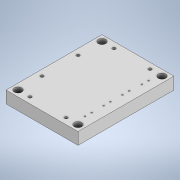
# Autodesk Inventor part: CasingBottomWithSlots
Saved by Autodesk Inventor 2020.4 (Build 244396010, 396A)
## iProperties
Created: 2021-10-02
Part Number: CasingBottomWithSlots
Material: Generic
Document SubType Name: Modeling
Designer: YUSTE
Density: 1 g/cm^3
Appearance: Default
Author: YUSTE
Autodesk Inventor part; units mm, degrees
ref_plane "YZ Plane" through (0, 0, 0) normal (1, 0, 0) x (0, 1, 0)
ref_plane "XZ Plane" through (0, 0, 0) normal (0, 1, 0) x (-1, 0, 0)
ref_plane "XY Plane" through (0, 0, 0) normal (0, 0, 1) x (1, 0, 0)
sketch "Sketch1" plane through (0, 0, 0) normal (0, 1, 0) x (-1, 0, 0)
  line L0 (0, 0) -> (152.4, 0)
  line L1 (152.4, 0) -> (152.4, 203.2)
  line L2 (152.4, 203.2) -> (0, 203.2)
  line L3 (0, 203.2) -> (0, 0)
  circle A0 centre (12.7, 190.5) radius 7.9375
  circle A1 centre (139.7, 190.5) radius 7.9375
  circle A2 centre (139.7, 12.7) radius 7.9375
  circle A3 centre (12.7, 12.7) radius 7.9375
  circle A4 centre (114.3, 190.5) radius 3.302
  circle A5 centre (38.1, 190.5) radius 3.302
  circle A6 centre (114.3, 12.7) radius 3.302
  circle A7 centre (38.1, 12.7) radius 3.302
  circle A8 centre (139.7, 139.7) radius 3.302
  circle A9 centre (139.7, 63.5) radius 3.302
  circle A10 centre (20.32, 168.148) radius 1.524
  circle A11 centre (20.32, 153.924) radius 1.524
  circle A12 centre (20.32, 128.524) radius 1.524
  circle A13 centre (20.32, 114.3) radius 1.524
  circle A14 centre (20.32, 88.9) radius 1.524
  circle A15 centre (20.32, 74.676) radius 1.524
  circle A16 centre (18.796, 49.276) radius 1.524
  circle A17 centre (18.796, 35.052) radius 1.524
  dimension "d0" = 152.4
  dimension "d1" = 203.2
  dimension "d40" = 15.875
  dimension "d41" = 15.875
  dimension "d42" = 15.875
  dimension "d43" = 15.875
  dimension "d44" = 12.7
  dimension "d45" = 12.7
  dimension "d46" = 12.7
  dimension "d47" = 12.7
  dimension "d48" = 12.7
  dimension "d49" = 12.7
  dimension "d50" = 12.7
  dimension "d51" = 12.7
  dimension "d52" = 177.8
  dimension "d53" = 127
  dimension "d54" = 6.604
  dimension "d55" = 6.604
  dimension "d56" = 25.4
  dimension "d57" = 25.4
  dimension "d58" = 12.7
  dimension "d59" = 12.7
  dimension "d60" = 6.604
  dimension "d61" = 6.604
  dimension "d62" = 12.7
  dimension "d63" = 12.7
  dimension "d64" = 25.4
  dimension "d65" = 25.4
  dimension "d66" = 6.604
  dimension "d67" = 6.604
  dimension "d68" = 50.8
  dimension "d69" = 50.8
  dimension "d70" = 12.7
  dimension "d71" = 12.7
  dimension "d72" = 3.048
  dimension "d73" = 3.048
  dimension "d74" = 3.048
  dimension "d75" = 3.048
  dimension "d76" = 3.048
  dimension "d77" = 3.048
  dimension "d78" = 20.32
  dimension "d79" = 20.32
  dimension "d80" = 20.32
  dimension "d81" = 20.32
  dimension "d82" = 20.32
  dimension "d83" = 20.32
  dimension "d84" = 22.352
  dimension "d85" = 14.224
  dimension "d86" = 25.4
  dimension "d87" = 14.224
  dimension "d88" = 25.4
  dimension "d89" = 14.224
  dimension "d90" = 3.048
  dimension "d91" = 3.048
  dimension "d92" = 25.4
  dimension "d93" = 14.224
  constraints: 18 centre point, 8 end point, 2 parallel, 1 horizontal, 1 perpendicular
  measures "d0" distance of L2.end L1.end
  measures "d1" distance of L1.end L0.end
  measures "d40" diameter of A0
  measures "d41" diameter of A1
  measures "d42" diameter of A2
  measures "d43" diameter of A3
  measures "d44" distance from line of L2 A0.centre
  measures "d45" distance from line of L3 A0.centre
  measures "d46" distance from line of L0 A3.centre
  measures "d47" distance from line of L3 A3.centre
  measures "d48" distance from line of L2 A1.centre
  measures "d49" distance from line of L1 A1.centre
  measures "d50" distance from line of L1 A2.centre
  measures "d51" distance from line of L0 A2.centre
  measures "d52" distance of A2.centre A1.centre
  measures "d53" distance of A0.centre A1.centre
  measures "d54" diameter of A4
  measures "d55" diameter of A5
  measures "d56" distance of A0.centre A5.centre
  measures "d57" distance of A1.centre A4.centre
  measures "d58" distance from line of L2 A4.centre
  measures "d59" distance from line of L2 A5.centre
  measures "d60" diameter of A6
  measures "d61" diameter of A7
  measures "d62" distance from line of L0 A7.centre
  measures "d63" distance from line of L0 A6.centre
  measures "d64" distance of A2.centre A6.centre
  measures "d65" distance of A3.centre A7.centre
  measures "d66" diameter of A8
  measures "d67" diameter of A9
  measures "d68" distance of A1.centre A8.centre
  measures "d69" distance of A2.centre A9.centre
  measures "d70" distance from line of L1 A8.centre
  measures "d71" distance from line of L1 A9.centre
  measures "d72" diameter of A10
  measures "d73" diameter of A11
  measures "d74" diameter of A12
  measures "d75" diameter of A13
  measures "d76" diameter of A14
  measures "d77" diameter of A15
  measures "d78" distance from line of L3 A10.centre
  measures "d79" distance from line of L3 A11.centre
  measures "d80" distance from line of L3 A12.centre
  measures "d81" distance from line of L3 A13.centre
  measures "d82" distance from line of L3 A14.centre
  measures "d83" distance from line of L3 A15.centre
  measures "d84" vertical distance of A10.centre A0.centre
  measures "d85" distance of A10.centre A11.centre
  measures "d86" distance of A11.centre A12.centre
  measures "d87" distance of A12.centre A13.centre
  measures "d88" distance of A14.centre A13.centre
  measures "d89" distance of A14.centre A15.centre
  measures "d90" diameter of A16
  measures "d91" diameter of A17
  measures "d92" vertical distance of A16.centre A15.centre
  measures "d93" distance of A16.centre A17.centre
extrude "Extrusion2" add sketch "Sketch1" along normal blind 25.4
body "Solid2"
